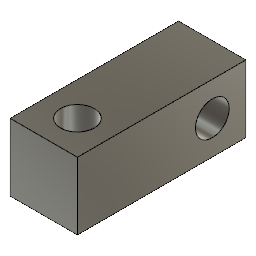
raspberry_pi_mount (Autodesk Fusion 360 design; units mm, degrees)
Autodesk Fusion 360 part; units mm, degrees
sketch "Sketch1" plane through (0, 0, 0) normal (0, 0, 1) x (1, 0, 0)
  line L0 (0, 0) -> (6, 0)
  line L1 (6, 0) -> (6, 15)
  line L2 (6, 15) -> (0, 15)
  line L3 (0, 15) -> (0, 0)
  circle A0 centre (3, 3) radius 1.5
  dimension "d1" = 6
  dimension "d2" = 15
  dimension "d3" = 3
  dimension "d4" = 3
  dimension "d5" = 3
  constraint horizontal L0
  constraint vertical L1
  constraint horizontal L2
  constraint vertical L3
  constraint coincident L0.start L3.end
  measures "d1" distance of L0.start L0.end
  measures "d2" distance of L0.start L2.end
  measures "d3" diameter of A0
  measures "d4" distance of L0 A0.centre
  measures "d5" distance of L1 A0.centre
extrude "Extrude1" add sketch "Sketch1" along normal blind 6
sketch "Sketch2" plane through (0, 0, 0) normal (-1, 0, 0) x (0, -1, 0)
  line L0 (-15, 0) -> (0, 0)
  line L1 (0, 0) -> (0, 6)
  line L2 (0, 6) -> (-15, 6)
  line L3 (-15, 6) -> (-15, 0)
  circle A0 centre (-12, 3) radius 1.5
  dimension "d8" = 3
  dimension "d9" = 3
  dimension "d10" = 3
  measures "d8" diameter of A0
  measures "d9" distance of L2 A0.centre
  measures "d10" distance of L3 A0.centre
extrude "Extrude2" cut sketch "Sketch2" against normal blind 6 contours A0
